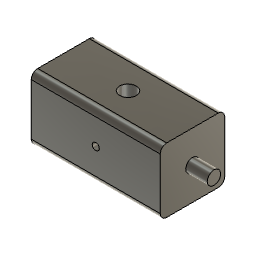
Rectangular holder (Autodesk Fusion 360 design; units mm, degrees)
Autodesk Fusion 360 part; units mm, degrees
sketch "Esquisse1" plane through (0, 0, 0) normal (0, 0, 1) x (1, 0, 0)
  line L0 (30.3919, -16.1268) -> (-29.6081, -16.1268)
  line L1 (-29.6081, -16.1268) -> (-29.6081, 13.8732)
  line L2 (-29.6081, 13.8732) -> (30.3919, 13.8732)
  line L3 (30.3919, 13.8732) -> (30.3919, -16.1268)
  dimension "d1" = 60
  dimension "d2" = 30
  constraint horizontal L0
  constraint vertical L1
  constraint horizontal L2
  constraint vertical L3
  measures "d1" distance of L0.start L0.end
  measures "d2" distance of L0.start L2.end
extrude "Extrusion1" add sketch "Esquisse1" along normal blind 30
sketch "Esquisse2" plane through (0, 0, 30) normal (0, 0, 1) x (-1, 0, 0)
  line L0 (-30.3919, -13.8732) -> (29.6081, -13.8732)
  line L1 (29.6081, -13.8732) -> (29.6081, 16.1268)
  line L2 (29.6081, 16.1268) -> (-30.3919, 16.1268)
  line L3 (-30.3919, 16.1268) -> (-30.3919, -13.8732)
  circle A0 centre (-0.3919, 1.1268) radius 3.75
  dimension "d5" = 7.5
  measures "d5" diameter of A0
extrude "Extrusion2" cut sketch "Esquisse2" against normal blind 30 contours A0
sketch "Esquisse3" plane through (0, 13.8732, 0) normal (0, 1, 0) x (-1, 0, 0)
  line L0 (-30.3919, 0) -> (29.6081, 0)
  line L1 (29.6081, 0) -> (29.6081, 30)
  line L2 (29.6081, 30) -> (-30.3919, 30)
  line L3 (-30.3919, 30) -> (-30.3919, 0)
  circle A0 centre (-0.3919, 15) radius 1.625
  dimension "d8" = 3.25
  measures "d8" diameter of A0
extrude "Extrusion3" cut sketch "Esquisse3" against normal blind 30 contours A0
sketch "Esquisse4" plane through (-29.6081, 0, 0) normal (-1, 0, 0) x (0, -1, 0)
  line L0 (-13.8732, 0) -> (16.1268, 0)
  line L1 (16.1268, 0) -> (16.1268, 30)
  line L2 (16.1268, 30) -> (-13.8732, 30)
  line L3 (-13.8732, 30) -> (-13.8732, 0)
  circle A0 centre (1.1268, 15) radius 5.5
  dimension "d11" = 11
  measures "d11" diameter of A0
extrude "Extrusion4" add sketch "Esquisse4" along normal blind 10 contours A0
delete_face "DeleteFace1" 2 faces at (-39.6081, 0.0561, 15.7248) (-36.2748, -6.62, 14.7258)
sketch "Esquisse5" plane through (-29.6081, 0, 0) normal (-1, 0, 0) x (0, -1, 0)
  line L0 (-13.8732, 0) -> (16.1268, 0)
  line L1 (16.1268, 0) -> (16.1268, 30)
  line L2 (16.1268, 30) -> (-13.8732, 30)
  line L3 (-13.8732, 30) -> (-13.8732, 0)
  circle A0 centre (1.1268, 15) radius 2.5
  dimension "d14" = 5
  measures "d14" diameter of A0
extrude "Extrusion5" add sketch "Esquisse5" along normal blind 10 contours A0
delete_face "DeleteFace2" 1 faces at (-36.2748, -3.6237, 14.8754)
sketch "Esquisse6" plane through (0, 0, 30) normal (0, 0, 1) x (-1, 0, 0)
  circle A0 centre (-0.3919, 1.1268) radius 3.75
  line L0 (-30.3919, -13.8732) -> (29.6081, -13.8732)
  line L1 (29.6081, -13.8732) -> (29.6081, 16.1268)
  line L2 (29.6081, 16.1268) -> (-30.3919, 16.1268)
  line L3 (-30.3919, 16.1268) -> (-30.3919, -13.8732)
extrude "Extrusion6" add sketch "Esquisse6" against normal blind 30 contours A0
sketch "Esquisse7" plane through (0, 0, 30) normal (0, 0, 1) x (-1, 0, 0)
  line L0 (-30.3919, -13.8732) -> (29.6081, -13.8732)
  line L1 (29.6081, -13.8732) -> (29.6081, 16.1268)
  line L2 (29.6081, 16.1268) -> (-30.3919, 16.1268)
  line L3 (-30.3919, 16.1268) -> (-30.3919, -13.8732)
  circle A0 centre (-0.3919, 1.1268) radius 3.86
  dimension "d19" = 7.72
  measures "d19" diameter of A0
extrude "Extrusion7" cut sketch "Esquisse7" against normal blind 30 contours A0
sketch "Esquisse8" plane through (-29.6081, 0, 0) normal (-1, 0, 0) x (0, -1, 0)
  line L0 (-13.8732, 0) -> (16.1268, 0)
  line L1 (16.1268, 0) -> (16.1268, 30)
  line L2 (16.1268, 30) -> (-13.8732, 30)
  line L3 (-13.8732, 30) -> (-13.8732, 0)
  circle A0 centre (1.1268, 15) radius 3.125
  dimension "d22" = 6.25
  measures "d22" diameter of A0
extrude "Extrusion8" add sketch "Esquisse8" along normal blind 10 contours A0
sketch "Esquisse9" plane through (30.3919, 0, 0) normal (1, 0, 0) x (0, 1, 0)
  line L0 (-16.1268, 0) -> (13.8732, 0)
  line L1 (13.8732, 0) -> (13.8732, 30)
  line L2 (13.8732, 30) -> (-16.1268, 30)
  line L3 (-16.1268, 30) -> (-16.1268, 0)
  circle A0 centre (-1.1268, 15) radius 3.125
  dimension "d25" = 6.25
  measures "d25" diameter of A0
extrude "Extrusion9" add sketch "Esquisse9" along normal blind 10 contours A0
fillet "Congé1" radius 3 1 edges at (0.3919, 13.8732, 30)
fillet "Congé2" radius 3 1 edges at (0.3919, -16.1268, 30)
fillet "Congé3" radius 3 1 edges at (0.3919, -16.1268, 0)
fillet "Congé4" radius 3 1 edges at (0.3919, 13.8732, 0)
